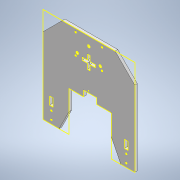
# Autodesk Inventor part: BoardProj
Saved by Autodesk Inventor 2020.1 (Build 241239000, 239)
## iProperties
Created: 2019-10-24
Part Number: BoardProj
Material: Generic
Document SubType Name: Modeling
Designer: j8qin
Density: 1 g/cm^3
Appearance: Default
Author: j8qin
Autodesk Inventor part; units mm, degrees
ref_plane "YZ Plane" through (0, 0, 0) normal (1, 0, 0) x (0, 1, 0)
ref_plane "XZ Plane" through (0, 0, 0) normal (0, 1, 0) x (-1, 0, 0)
ref_plane "XY Plane" through (0, 0, 0) normal (0, 0, 1) x (1, 0, 0)
sketch "Sketch1" plane through (0, 0, 0) normal (0, 0, 1) x (1, 0, 0)
  line L0 (-88.9, -92.075) -> (-88.9, 92.075)
  line L1 (-88.9, 92.075) -> (88.9, 92.075)
  line L2 (88.9, 92.075) -> (88.9, -92.075)
  line L3 (88.9, -92.075) -> (-88.9, -92.075)
  line L4 (-88.9, -92.075) -> (88.9, 92.075) construction
  line L5 (-88.9, 92.075) -> (88.9, -92.075) construction
  line L6 (-2.54, 53.34) -> (2.54, 53.34) construction
  line L7 (2.54, 78.74) -> (-2.54, 78.74) construction
  line L8 (-12.7, 63.5) -> (-12.7, 68.58) construction
  line L9 (12.7, 68.58) -> (12.7, 63.5) construction
  line L10 (-2.54, 63.5) -> (-12.7, 63.5) construction
  line L11 (-2.54, 63.5) -> (-2.54, 53.34) construction
  line L12 (-2.54, 78.74) -> (-2.54, 68.58) construction
  line L13 (-12.7, 68.58) -> (-2.54, 68.58) construction
  line L14 (2.54, 68.58) -> (12.7, 68.58) construction
  line L15 (12.7, 63.5) -> (2.54, 63.5) construction
  line L16 (2.54, 53.34) -> (2.54, 63.5) construction
  line L17 (2.54, 68.58) -> (2.54, 78.74) construction
  circle A0 centre (25.4, 85.725) radius 1.4605
  line L18 (12.7, 66.04) -> (-12.7, 66.04) construction
  line L19 (0, 53.34) -> (0, 78.74) construction
  circle A1 centre (25.4, 46.355) radius 1.4605
  circle A2 centre (-25.4, 85.725) radius 1.4605
  circle A3 centre (-25.4, 46.355) radius 1.4605
  line L20 (12.7, 50.165) -> (-12.7, 50.165)
  line L21 (-12.7, 50.165) -> (-12.7, 45.085)
  line L22 (-12.7, 45.085) -> (12.7, 45.085)
  line L23 (12.7, 45.085) -> (12.7, 50.165)
  line L24 (12.7, 50.165) -> (-12.7, 45.085) construction
  line L25 (-12.7, 50.165) -> (12.7, 45.085) construction
  line L26 (2.54, 60.325) -> (-2.54, 60.325)
  line L27 (-2.54, 60.325) -> (-2.54, 34.925)
  line L28 (-2.54, 34.925) -> (2.54, 34.925)
  line L29 (2.54, 34.925) -> (2.54, 60.325)
  line L30 (2.54, 60.325) -> (-2.54, 34.925) construction
  line L31 (-2.54, 60.325) -> (2.54, 34.925) construction
  circle A4 centre (22.225, 52.4607) radius 2.4384 projected
  circle A5 centre (0, 74.6857) radius 2.4384 projected
  circle A6 centre (-22.225, 52.4607) radius 2.4384 projected
  line L32 (7.62, -36.5282) -> (12.7, -36.5282) projected
  line L33 (12.7, -36.5282) -> (12.7, -11.1282) projected
  line L34 (12.7, -11.1282) -> (12.7, -6.2879) projected
  line L35 (7.62, -6.2879) -> (12.7, -6.2879) projected
  line L36 (2.54, -6.2879) -> (7.62, -6.2879) projected
  line L37 (-2.54, -6.2879) -> (2.54, -6.2879) projected
  line L38 (-7.62, -6.2879) -> (-2.54, -6.2879) projected
  line L39 (-7.62, -11.1282) -> (-7.62, -6.2879) projected
  line L40 (-7.62, -36.5282) -> (-7.62, -11.1282) projected
  line L41 (-2.54, -36.5282) -> (2.54, -36.5282) projected
  line L42 (-7.62, -36.5282) -> (-2.54, -36.5282) projected
  line L43 (2.54, -36.5282) -> (7.62, -36.5282) projected
  line L44 (15.24, -3.7479) -> (15.24, -11.1282)
  line L45 (15.24, -11.1282) -> (15.24, -39.0682)
  line L46 (15.24, -39.0682) -> (7.62, -39.0682)
  line L47 (7.62, -39.0682) -> (2.54, -39.0682)
  line L48 (2.54, -39.0682) -> (-2.54, -39.0682)
  line L49 (-2.54, -39.0682) -> (-10.16, -39.0682)
  line L50 (-10.16, -39.0682) -> (-10.16, -11.1282)
  line L51 (-10.16, -11.1282) -> (-10.16, -3.7479)
  line L52 (-10.16, -3.7479) -> (-2.54, -3.7479)
  line L53 (-2.54, -3.7479) -> (2.54, -3.7479)
  line L54 (2.54, -3.7479) -> (7.62, -3.7479)
  line L55 (7.62, -3.7479) -> (15.24, -3.7479)
  line L56 (-38.1, -27.758) -> (43.18, -27.758)
  line L57 (43.18, -27.758) -> (43.18, -15.058)
  line L58 (43.18, -15.058) -> (-38.1, -15.058)
  line L59 (-38.1, -15.058) -> (-38.1, -27.758)
  line L60 (-38.1, -27.758) -> (43.18, -15.058) construction
  line L61 (43.18, -27.758) -> (-38.1, -15.058) construction
  line L62 (-38.1, -27.758) -> (-38.1, -92.075)
  line L63 (43.18, -27.758) -> (43.18, -92.075)
  point P0 (0, 0)
  point P1 (0, 47.625)
  point P2 (2.54, 50.165)
  point P3 (2.54, 45.085)
  point P4 (-2.54, 45.085)
  point P5 (-2.54, 50.165)
  point P6 (2.54, -21.408)
  point P7 (2.54, -21.408)
  point P8 (-10.16, -27.758)
  point P9 (-10.16, -15.058)
  point P10 (15.24, -15.058)
  point P11 (15.24, -27.758)
  dimension "d0" = 184.15
  dimension "d1" = 177.8
  dimension "d26" = 5.08
  dimension "d27" = 5.08
  dimension "d28" = 6.35
  dimension "d29" = 2.921
  dimension "d30" = 63.5
  dimension "d31" = 25.4
  dimension "d32" = 25.4
  dimension "d33" = 25.4
  dimension "d34" = 5.08
  dimension "d35" = 5.08
  dimension "d36" = 44.45
  dimension "d37" = 88.9
  dimension "d40" = 2.54
  dimension "d41" = 81.28
  dimension "d42" = 12.7
  dimension "d43" = 30.2403
  dimension "d44" = 15.1201
  constraints: 104 end point, 18 parallel, 13 midpoint, 10 perpendicular, 6 horizontal, 4 centre point, 3 symmetric about line, 2 point on line, 1 vertical, 1 vertical alignment, 14 other
  measures "d0" distance of L0.start L0.end
  measures "d1" distance of L0.end L1.end
  measures "d26" distance of L8.start L8.end
  measures "d27" distance of L7.start L7.end
  measures "d28" distance from line of L1 A0.centre
  measures "d29" diameter of A0
  measures "d30" distance from line of L2 A0.centre
  measures "d31" distance between parallel lines of L7 L6
  measures "d32" distance of L20.start L20.end
  measures "d33" distance of L26.end L27.end
  measures "d34" distance of L20.end L21.end
  measures "d35" distance of L26.start L26.end
  measures "d36" distance from line of L1 point (0, 47.625)
  measures "d37" distance from line of L0 point (0, 47.625)
  measures "d40" distance between parallel lines of L34 L44
  measures "d41" distance of L56.start L56.end
  measures "d42" distance of L56.end L57.end
  measures "d43" distance between parallel lines of L32 L35
  measures "d44" distance from line of L32 point (2.54, -21.408)
extrude "Extrusion1" add sketch "Sketch1" along normal mid plane 5.08 contours L0 L1 L2 L3 L63 L57 L58 L45 L44 L55 L54 L53 L52 L51 L50 L59 L62
sketch "Sketch2" plane through (0, 0, 2.54) normal (0, 0, 1) x (1, 0, 0)
  circle A0 centre (-22.86, -3.175) radius 1.4605 construction
  circle A1 centre (-12.7, -3.175) radius 1.4605 construction
  line L0 (0, -6.35) -> (0, 0) construction
  line L1 (-25.4, 0) -> (0, 0) construction
  line L2 (-25.4, 0) -> (-25.4, -6.35) construction
  line L3 (0, -6.35) -> (-25.4, -6.35) construction
  line L4 (15.24, -6.35) -> (15.24, 0) construction
  line L5 (0, 0) -> (15.24, 0) construction
  line L6 (0, -6.35) -> (0, 0) construction
  line L7 (15.24, -6.35) -> (0, -6.35) construction
  line L8 (69.088, -61.595) -> (69.088, -46.355)
  line L9 (69.088, -46.355) -> (75.438, -46.355)
  line L10 (75.438, -46.355) -> (75.438, -61.595)
  line L11 (75.438, -86.995) -> (69.088, -86.995) construction
  line L12 (88.9, -92.075) -> (88.9, 92.075) projected
  line L13 (-88.9, -92.075) -> (88.9, -92.075) projected
  line L14 (69.088, -61.595) -> (75.438, -61.595)
  circle A2 centre (72.263, -84.455) radius 1.4605
  circle A3 centre (72.263, -69.215) radius 1.4605
  point P0 (-25.4, -3.175)
  dimension "d14" = 13.462
  dimension "d15" = 6.35
  dimension "d16" = 5.08
  dimension "d17" = 40.64
  dimension "d18" = 15.24
  dimension "d19" = 2.921
  dimension "d20" = 2.921
  dimension "d21" = 15.24
  dimension "d22" = 3.175
  dimension "d23" = 2.54
  constraints: 26 end point, 4 centre point, 4 perpendicular, 1 vertical, 1 vertical alignment
  measures "d14" distance between parallel lines of L12 L10
  measures "d15" distance of L11.start L11.end
  measures "d16" distance between parallel lines of L13 L11
  measures "d17" distance of L11.end L8.end
  measures "d18" distance between parallel lines of L9 L14
  measures "d19" diameter of A2
  measures "d20" diameter of A3
  measures "d21" distance of A2.centre A3.centre
  measures "d22" distance from line of L8 A2.centre
  measures "d23" distance from line of L11 A2.centre
extrude "Extrusion2" cut sketch "Sketch2" against normal through all
mirror "Mirror1" about plane through (0, 0, 0) normal (1, 0, 0) of "Extrusion2"
sketch "Sketch7" plane through (0, 0, 2.54) normal (0, 0, 1) x (1, 0, 0)
  circle A0 centre (-72.263, -84.455) radius 1.4605 projected
  line L0 (-69.088, -61.595) -> (-75.438, -61.595) projected
  line L1 (-75.438, -61.595) -> (-75.438, -46.355) projected
  line L2 (-75.438, -46.355) -> (-69.088, -46.355) projected
  line L3 (-69.088, -46.355) -> (-69.088, -61.595) projected
  circle A1 centre (-72.263, -69.215) radius 1.4605 projected
  circle A2 centre (72.263, -84.455) radius 1.4605 projected
  circle A3 centre (72.263, -69.215) radius 1.4605 projected
  line L4 (69.088, -46.355) -> (75.438, -46.355) projected
  line L5 (75.438, -46.355) -> (75.438, -61.595) projected
  line L6 (75.438, -61.595) -> (69.088, -61.595) projected
  line L7 (69.088, -61.595) -> (69.088, -46.355) projected
  line L8 (15.24, -3.7479) -> (15.24, -15.058) projected
  line L9 (15.24, -15.058) -> (43.18, -15.058) projected
  line L10 (43.18, -15.058) -> (43.18, -92.075) projected
  line L11 (-10.16, -15.058) -> (-10.16, -3.7479) projected
  line L12 (-38.1, -92.075) -> (-38.1, -15.058) projected
  line L13 (-38.1, -15.058) -> (-10.16, -15.058) projected
  line L14 (-10.16, -3.7479) -> (15.24, -3.7479) projected
  circle A4 centre (-22.225, 52.4607) radius 2.4384 projected
  circle A5 centre (0, 74.6857) radius 2.4384 projected
  circle A6 centre (22.225, 52.4607) radius 2.4384 projected
  circle A7 centre (25.4, 85.725) radius 1.4605 projected
  circle A8 centre (25.4, 46.355) radius 1.4605 projected
  circle A9 centre (-25.4, 85.725) radius 1.4605 projected
  circle A10 centre (-25.4, 46.355) radius 1.4605 projected
  line L15 (-12.7, 45.085) -> (-12.7, 50.165) projected
  line L16 (-12.7, 50.165) -> (-2.54, 50.165) projected
  line L17 (-2.54, 50.165) -> (-2.54, 60.325) projected
  line L18 (-2.54, 60.325) -> (2.54, 60.325) projected
  line L19 (2.54, 60.325) -> (2.54, 50.165) projected
  line L20 (2.54, 50.165) -> (12.7, 50.165) projected
  line L21 (12.7, 50.165) -> (12.7, 45.085) projected
  line L22 (12.7, 45.085) -> (2.54, 45.085) projected
  line L23 (2.54, 45.085) -> (2.54, 34.925) projected
  line L24 (2.54, 34.925) -> (-2.54, 34.925) projected
  line L25 (-2.54, 34.925) -> (-2.54, 45.085) projected
  line L26 (-2.54, 45.085) -> (-12.7, 45.085) projected
  line L27 (-88.9, -92.075) -> (-38.1, -92.075) projected
  line L28 (88.9, -92.075) -> (88.9, 92.075) projected
  line L29 (88.9, 92.075) -> (-88.9, 92.075) projected
  line L30 (-88.9, 92.075) -> (-88.9, -92.075) projected
  line L31 (43.18, -92.075) -> (88.9, -92.075) projected
  point P0 (0, 0)
sketch "Sketch8" plane through (0, 0, 2.54) normal (0, 0, 1) x (1, 0, 0)
  line L0 (-57.15, -92.075) -> (-38.1, -53.975)
  line L1 (0, 0) -> (0, -92.075) construction
  line L2 (-88.9, -92.075) -> (-38.1, -92.075) projected
  line L3 (-38.1, -92.075) -> (-38.1, -15.058) projected
  line L4 (-57.15, -92.075) -> (-38.1, -92.075)
  line L5 (43.18, -15.058) -> (43.18, -92.075) projected
  line L6 (43.18, -92.075) -> (62.23, -92.075)
  line L7 (43.18, -92.075) -> (88.9, -92.075) projected
  line L8 (62.23, -92.075) -> (43.18, -53.975)
  line L9 (43.18, -53.975) -> (43.18, -92.075)
  dimension "d45" = 19.05
  dimension "d46" = 38.1
  dimension "d47" = 19.05
  dimension "d48" = 38.1
  constraints: 12 end point, 3 point on line, 1 horizontal, 1 perpendicular, 1 vertical
  measures "d45" distance of L2.end L0.start
  measures "d46" distance of L2.end L0.end
  measures "d47" distance of L5.end L6.end
  measures "d48" distance of L5.end L8.end
extrude "Extrusion3" cut sketch "Sketch8" against normal blind 25.4
sketch "Sketch9" plane through (0, 0, 2.54) normal (0, 0, 1) x (1, 0, 0)
  line L0 (-88.9, 92.075) -> (88.9, 92.075) projected
  line L1 (50.8, 92.075) -> (88.9, 53.975)
  line L2 (88.9, 53.975) -> (88.9, 92.075)
  line L3 (88.9, 92.075) -> (50.8, 92.075)
  line L4 (-88.9, -92.075) -> (-88.9, 92.075) projected
  line L5 (-88.9, 92.075) -> (-88.9, 53.975)
  line L6 (-50.8, 92.075) -> (-88.9, 53.975)
  line L7 (-88.9, 92.075) -> (-50.8, 92.075)
  point P0 (0, 0)
  dimension "d51" = 38.1
  dimension "d52" = 38.1
  dimension "d53" = 38.1
  constraints: 12 end point, 3 point on line, 2 collinear, 2 perpendicular
  measures "d51" distance of L0.end L1.start
  measures "d52" distance of L0.end L1.end
  measures "d53" distance of L0.start L6.start
extrude "Extrusion4" cut sketch "Sketch9" against normal blind 25.4
equation "\"d44\" = 0.5 * d43"
body "Solid1"
